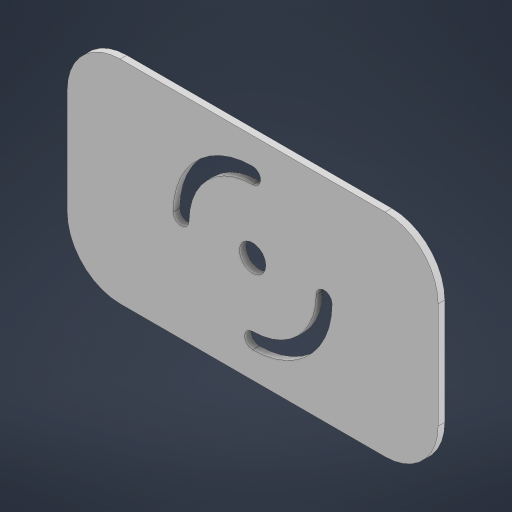
# Autodesk Inventor part: Front_plate
Saved by Autodesk Inventor 2024 (Build 280153000, 153)
## iProperties
Created: 2024-02-08
Part Number: Front_plate
Material: Generic
Document SubType Name: Modeling
Designer: calvi
Density: 1 g/cm^3
Appearance: Default
Author: calvi
Autodesk Inventor part; units mm, degrees
ref_plane "YZ Plane" through (0, 0, 0) normal (1, 0, 0) x (0, 1, 0)
ref_plane "XZ Plane" through (0, 0, 0) normal (0, 1, 0) x (-1, 0, 0)
ref_plane "XY Plane" through (0, 0, 0) normal (0, 0, 1) x (1, 0, 0)
sketch "Sketch1" plane through (0, 0, 0) normal (0, 0, 1) x (1, 0, 0)
  line L0 (0, 0) -> (177.8, 0)
  line L1 (177.8, 0) -> (177.8, 101.6)
  line L2 (177.8, 101.6) -> (0, 101.6)
  line L3 (0, 101.6) -> (0, 0)
  arc A0 (25.4, 101.6) -> (0, 76.2) centre (25.4, 76.2) ccw
  arc A1 (177.8, 76.2) -> (152.4, 101.6) centre (152.4, 76.2) ccw
  arc A2 (152.4, 0) -> (177.8, 25.4) centre (152.4, 25.4) ccw
  arc A3 (0, 25.4) -> (25.4, 0) centre (25.4, 25.4) ccw
  circle A4 centre (88.9, 50.8) radius 6.35
  arc A5 (88.9, 85.09) -> (54.61, 50.8) centre (88.9, 50.8) ccw construction
  arc A6 (88.9, 88.9) -> (50.8, 50.8) centre (88.9, 50.8) ccw
  arc A7 (88.9, 81.28) -> (58.42, 50.8) centre (88.9, 50.8) ccw
  arc A8 (88.9, 81.28) -> (88.9, 88.9) centre (88.9, 85.09) ccw
  arc A9 (50.8, 50.8) -> (58.42, 50.8) centre (54.61, 50.8) ccw
  line L4 (88.9, 50.8) -> (54.61, 50.8) construction
  line L5 (88.9, 50.8) -> (88.9, 85.09) construction
  arc A10 (88.9, 20.32) -> (119.38, 50.8) centre (88.9, 50.8) ccw
  line L6 (88.9, 50.8) -> (123.19, 50.8) construction
  arc A11 (88.9, 16.51) -> (123.19, 50.8) centre (88.9, 50.8) ccw construction
  arc A12 (127, 50.8) -> (119.38, 50.8) centre (123.19, 50.8) ccw
  arc A13 (88.9, 12.7) -> (127, 50.8) centre (88.9, 50.8) ccw
  arc A14 (88.9, 20.32) -> (88.9, 12.7) centre (88.9, 16.51) ccw
  point P0 (0, 0)
  dimension "d2" = 177.8
  dimension "d3" = 101.6
  dimension "d4" = 50.8
  dimension "d5" = 50.8
  dimension "d6" = 50.8
  dimension "d7" = 50.8
  dimension "d8" = 12.7
  dimension "d9" = 50.8
  dimension "d10" = 88.9
  dimension "d11" = 34.29
  dimension "d12" = 90
  dimension "d13" = 7.62
  dimension "d14" = 360
  dimension "d15" = 0
  dimension "d16" = 0
  constraints: 28 point on circle, 15 centre point, 14 end point, 12 tangent, 8 point on line, 2 parallel, 1 coincident, 1 horizontal, 1 perpendicular, 1 vertical, 27 other
  measures "d2" distance of L2.end L1.end
  measures "d3" distance of L1.end L0.end
  measures "d4" diameter of A0
  measures "d5" diameter of A1
  measures "d6" diameter of A2
  measures "d7" diameter of A3
  measures "d8" diameter of A4
  measures "d9" distance from line of L0 A4.centre
  measures "d10" distance from line of L1 A4.centre
  measures "d11" radius of A5
  measures "d12" angle of L5 L4
  measures "d13" diameter of A9
  measures "d15" distance of point (0, 0) L0.start
  measures "d16" distance of L0.start point (0, 0)
extrude "Extrusion1" add sketch "Sketch1" along normal blind 3.175 contours A3 L3 A0 L2 A1 L1 A2 L0
body "Solid1"
